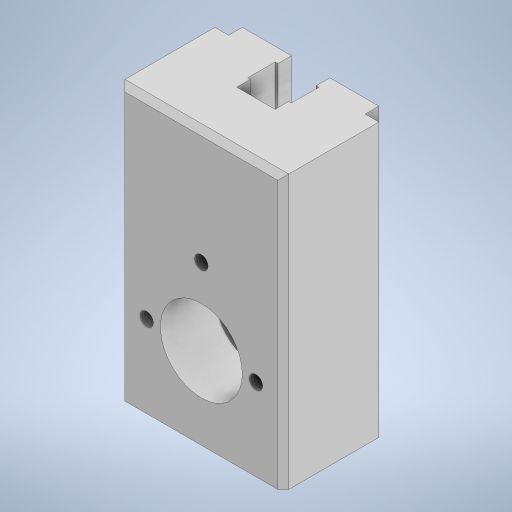
# Autodesk Inventor part: Schneidführung
Saved by Autodesk Inventor 2024 (Build 280153000, 153)
## iProperties
Created: 2023-05-12
Part Number: Schneidführung
Material: Generic
Document SubType Name: Modeling
Designer: Raj
Density: 1 g/cm^3
Appearance: Default
Author: Raj
Autodesk Inventor part; units mm, degrees
ref_plane "YZ Plane" through (0, 0, 0) normal (1, 0, 0) x (0, 1, 0)
ref_plane "XZ Plane" through (0, 0, 0) normal (0, 1, 0) x (-1, 0, 0)
ref_plane "XY Plane" through (0, 0, 0) normal (0, 0, 1) x (1, 0, 0)
sketch "Sketch1" plane through (0, 0, 0) normal (0, 0, 1) x (1, 0, 0)
  line L0 (0, 35) -> (0, 0)
  line L1 (0, 0) -> (-60, 0)
  line L2 (-60, 0) -> (-60, 35)
  line L3 (-60, 40) -> (0, 0) construction
  line L4 (0, 40) -> (-60, 0) construction
  line L5 (-55, 40) -> (-55, 35)
  line L6 (-55, 35) -> (-60, 35)
  line L7 (-5, 40) -> (-5, 35)
  line L8 (-5, 35) -> (0, 35)
  line L9 (-37, 40) -> (-37, 35)
  line L10 (-37, 35) -> (-38, 35)
  line L11 (-38, 35) -> (-38, 25)
  line L12 (-38, 25) -> (-37, 25)
  line L13 (-37, 25) -> (-37, 20)
  line L14 (-37, 20) -> (-23, 20)
  line L15 (-23, 20) -> (-23, 25)
  line L16 (-23, 25) -> (-22, 25)
  line L17 (-22, 25) -> (-22, 35)
  line L18 (-22, 35) -> (-23, 35)
  line L19 (-23, 35) -> (-23, 40)
  line L20 (-55, 40) -> (-37, 40)
  line L21 (-23, 40) -> (-5, 40)
  point P0 (-30, 20)
  dimension "d1" = 60
  dimension "d2" = 5
  dimension "d3" = 5
  dimension "d4" = 5
  dimension "d5" = 5
  dimension "d7" = 90
  dimension "d8" = 5
  dimension "d9" = 1
  dimension "d10" = 10
  dimension "d11" = 1
  dimension "d12" = 5
  dimension "d13" = 14
  dimension "d14" = 5
  dimension "d15" = 1
  dimension "d16" = 10
  dimension "d17" = 1
  dimension "d18" = 5
  dimension "d19" = 7
  dimension "d20" = 16
  dimension "d21" = 40
  dimension "d22" = 23
  dimension "d23" = 40
  dimension "d24" = 67.38
  constraints: 44 end point, 11 perpendicular, 6 point on line, 3 parallel, 2 horizontal, 2 midpoint
  measures "d1" distance from line of L0.end L2
  measures "d2" distance of L2.end L5.end
  measures "d3" distance of L5.start L5.end
  measures "d4" distance of L0.start L7.end
  measures "d5" distance of L7.start L7.end
  measures "d7" angle of L2 L6
  measures "d8" distance of L9.start L9.end
  measures "d9" distance of L9.end L10.end
  measures "d10" distance of L10.end L11.end
  measures "d11" distance of L11.end L12.end
  measures "d12" distance of L12.end L13.end
  measures "d13" distance of L13.end L14.end
  measures "d14" distance of L14.end L15.end
  measures "d15" distance of L15.end L16.end
  measures "d16" distance of L16.end L17.end
  measures "d17" distance of L17.end L18.end
  measures "d18" distance of L18.end L19.end
  measures "d19" distance from line of L9 point (-30, 20)
  measures "d20" distance between parallel lines of L17 L11
  measures "d21" distance between parallel lines of L1 L20
  measures "d22" distance from line of L0.end L15
  measures "d23" distance from line of L0.end L21
  measures "d24" angle of L3 L4
extrude "Extrusion1" add sketch "Sketch1" against normal blind 100
sketch "Sketch2" plane through (0, 0, -100) normal (0, 0, -1) x (-1, 0, 0)
  line L0 (0, 0) -> (60, 0) projected
  line L1 (0, 35) -> (0, 0) projected
  point P0 (20, 10)
  point P1 (40, 10)
  dimension "d27" = 10
  dimension "d28" = 10
  dimension "d29" = 20
  dimension "d30" = 20
  measures "d27" distance from line of point (20, 10) L0
  measures "d28" distance from line of L0 point (40, 10)
  measures "d29" distance from line of point (20, 10) L1
  measures "d30" distance of point (40, 10) point (20, 10)
hole "Hole1" at (-20, 10, -100) at (-40, 10, -100) direction (0, 0, 1) diameter 6.647 depth 15 tip angle 118 thread size "M8x1.25" class "6H" standard "ISO Metric profile"
sketch "Sketch3" plane through (-60, 0, 0) normal (0, -1, 0) x (1, 0, 0)
  circle A0 centre (30, -70) radius 15
  line L0 (60, -100) -> (0, -100) projected
  line L1 (60, 0) -> (60, -100) projected
  dimension "d38" = 30
  dimension "d41" = 30
  dimension "d42" = 30
  constraints: 1 centre point
  measures "d38" diameter of A0
  measures "d41" distance from line of A0.centre L0
  measures "d42" distance from line of L1 A0.centre
extrude "Extrusion2" cut sketch "Sketch3" against normal blind 20
sketch "Sketch4" plane through (-60, 0, 0) normal (0, -1, 0) x (1, 0, 0)
  line L0 (0, 0) -> (0, -100) projected
  line L1 (60, -100) -> (0, -100) projected
  point P0 (60, 0)
  point P1 (30, -42)
  point P2 (50, -70)
  point P3 (10, -70)
  dimension "d43" = 30
  dimension "d44" = 58
  dimension "d45" = 30
  dimension "d46" = 30
  dimension "d47" = 40
  dimension "d48" = 10
  measures "d43" distance from line of L0 point (30, -42)
  measures "d44" distance from line of L1 point (30, -42)
  measures "d45" distance from line of L1 point (10, -70)
  measures "d46" distance from line of L1 point (50, -70)
  measures "d47" distance of point (10, -70) point (50, -70)
  measures "d48" distance from line of L0 point (10, -70)
hole "Hole2" at (-30, 0, -42) at (-10, 0, -70) at (-50, 0, -70) direction (0, 1, 0) diameter 4.917 depth 10 tip angle 118 thread size "M6x1" class "6H" standard "ISO Metric profile"
sketch "Sketch5" plane through (-55, 40, 0) normal (0, 1, 0) x (1, 0, 0)
  line L0 (0, 100) -> (18, 100) projected
  line L1 (-5, 0) -> (-5, 100) projected
  point P0 (55, 0)
  point P1 (8, 85)
  point P2 (8, 50)
  point P3 (8, 15)
  point P4 (42, 85)
  point P5 (42, 50)
  point P6 (42, 15)
  dimension "d37" = 118
  dimension "d56" = 15
  dimension "d57" = 13
  dimension "d60" = 35
  dimension "d63" = 34
  constraints: 1 horizontal, 1 vertical, 5 other
  measures "d56" distance from line of point (8, 85) L0
  measures "d57" distance from line of point (8, 85) L1
  measures "d60" distance of point (8, 85) point (8, 50)
  measures "d63" distance of point (8, 85) point (42, 85)
hole "Hole3" at (-47, 40, -85) at (-47, 40, -50) at (-47, 40, -15) at (-13, 40, -85) at (-13, 40, -50) at (-13, 40, -15) direction (0, -1, 0) diameter 4.917 depth 12 tip angle 118 thread size "M6x1" class "6H" standard "ISO Metric profile"
chamfer "Chamfer1" distance 2 angle 45 3 edges at (0, 0, -50) (-60, 0, -50) (-30, 0, 0)
body "Solid1"
